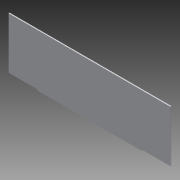
# Autodesk Inventor part: electronics board
Saved by Autodesk Inventor 2012 (Build 160160000, 160)
## iProperties
Created: 2013-10-01
Part Number: electronics board
Material: Default
Document SubType Name: Modeling
Designer: Bryce
Density: 1 g/cm^3
Author: Bryce
Autodesk Inventor part; units mm, degrees
ref_plane "YZ Plane" through (0, 0, 0) normal (1, 0, 0) x (0, 1, 0)
ref_plane "XZ Plane" through (0, 0, 0) normal (0, 1, 0) x (-1, 0, 0)
ref_plane "XY Plane" through (0, 0, 0) normal (0, 0, 1) x (1, 0, 0)
sketch "Sketch1" plane through (0, 0, 0) normal (0, 0, 1) x (1, 0, 0)
  line L0 (0, 0) -> (165.1, 0) construction
  line L1 (939.8, 0) -> (939.8, 6.35) construction
  line L2 (939.8, 304.8) -> (0, 304.8)
  line L3 (0, 304.8) -> (0, 6.35)
  line L4 (0, 6.35) -> (165.1, 6.35)
  line L5 (165.1, 6.35) -> (165.1, 0)
  line L6 (939.8, 6.35) -> (774.7, 6.35)
  line L7 (774.7, 6.35) -> (774.7, 0)
  line L8 (0, 6.35) -> (0, 0) construction
  line L9 (165.1, 0) -> (774.7, 0)
  line L10 (774.7, 0) -> (939.8, 0) construction
  line L11 (939.8, 6.35) -> (939.8, 304.8)
  dimension "d0" = 304.8
  dimension "d1" = 939.8
  dimension "d2" = 165.1
  dimension "d3" = 6.35
  constraints: 24 end point, 13 perpendicular, 7 parallel, 3 horizontal, 2 collinear, 1 point on line
  measures "d0" distance of L2.end L0.start
  measures "d1" distance of L0.start L1.start
  measures "d2" distance of L3.end L4.end
  measures "d3" distance of L4.end L0.end
extrude "Extrusion1" add sketch "Sketch1" along normal blind 6.35
body "Solid1"
